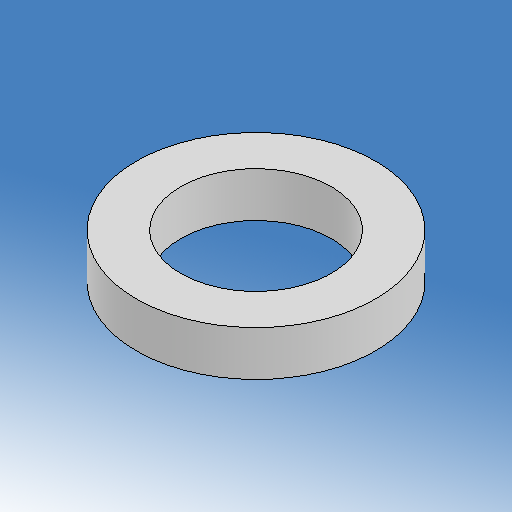
# Autodesk Inventor part: 8mKeyyedShaftSpacer_BevelToSpurShaft
Saved by Autodesk Inventor 2025 (Build 290162000, 162)
## iProperties
Created: 2024-06-12
Part Number: 8mKeyyedShaftSpacer_BevelToSpurShaft
Material: Generic
Document SubType Name: Modeling
Designer: seene
Density: 1 g/cm^3
Appearance: Default
Author: seene
Autodesk Inventor part; units mm, degrees
ref_plane "YZ Plane" through (0, 0, 0) normal (1, 0, 0) x (0, 1, 0)
ref_plane "XZ Plane" through (0, 0, 0) normal (0, 1, 0) x (-1, 0, 0)
ref_plane "XY Plane" through (0, 0, 0) normal (0, 0, 1) x (1, 0, 0)
sketch "Sketch1" plane through (0, 0, 0) normal (0, 1, 0) x (-1, 0, 0)
  circle A0 centre (0, 0) radius 4.25
  circle A1 centre (0, 0) radius 6.75
  line L0 (0, 0) -> (-4.25, 0) construction
  point P0 (4.1833, 0.75)
  dimension "d1" = 2.5
  constraints: 2 centre point, 2 end point, 2 point on circle, 1 coincident, 1 horizontal
  measures "d1" radial gap between concentric circles of A0 A1
extrude "Extrusion1" add sketch "Sketch1" along normal blind 2.54
body "Solid1"
